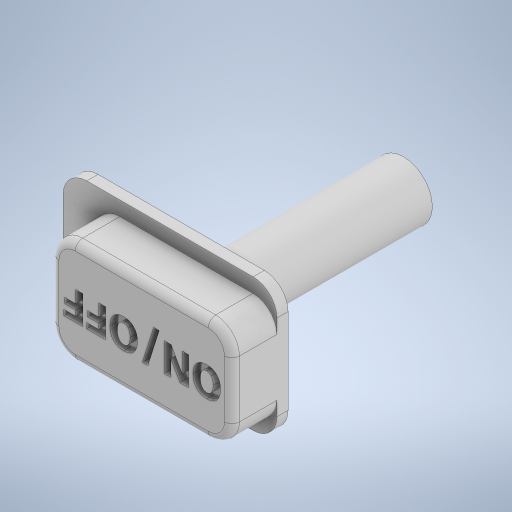
# Autodesk Inventor part: Button Cover
Saved by Autodesk Inventor 2023 (Build 270158000, 158)
## iProperties
Created: 2024-03-21
Part Number: Button Cover
Material: Generic
Document SubType Name: Modeling
Designer: Pobe Tran
Density: 1 g/cm^3
Appearance: Default
Author: Pobe Tran
Autodesk Inventor part; units mm, degrees
ref_plane "YZ Plane" through (0, 0, 0) normal (1, 0, 0) x (0, 1, 0)
ref_plane "XZ Plane" through (0, 0, 0) normal (0, 1, 0) x (-1, 0, 0)
ref_plane "XY Plane" through (0, 0, 0) normal (0, 0, 1) x (1, 0, 0)
sketch "Sketch1" plane through (0, 0, 0) normal (0, 0, 1) x (1, 0, 0)
  circle A0 centre (0, 0) radius 1.75 projected
  circle A1 centre (0, 0) radius 3.85
  point P0 (0, 0)
  constraints: 1 centre point
extrude "Extrusion1" add sketch "Sketch1" against normal blind 5
sketch "Sketch2" plane through (0, 0, 0) normal (0, 0, 1) x (1, 0, 0)
  point P0 (0, 0)
sketch "Sketch3" plane through (0, 0, 0) normal (0, 0, 1) x (1, 0, 0)
  circle A0 centre (0, 0) radius 3.85
  constraints: 1 centre point, 1 coincident
extrude "Extrusion2" add sketch "Sketch3" along normal blind 22.5
sketch "Sketch4" plane through (0, 0, 22.5) normal (0, 0, 1) x (1, 0, 0)
  line L0 (12.065, -6.985) -> (-12.065, -6.985)
  line L1 (-12.065, -6.985) -> (-12.065, 6.985)
  line L2 (-12.065, 6.985) -> (12.065, 6.985)
  line L3 (12.065, 6.985) -> (12.065, -6.985)
  circle A0 centre (0, 0) radius 1.85 projected
  line L4 (12.065, -6.985) -> (-12.065, 6.985) construction
  line L5 (-12.065, -6.985) -> (12.065, 6.985) construction
  line L6 (12.065, 12.065) -> (-12.065, 12.065) construction
  line L7 (-12.065, 12.065) -> (-12.065, 26.035) construction
  line L8 (-12.065, 26.035) -> (12.065, 26.035) construction
  line L9 (12.065, 26.035) -> (12.065, 12.065) construction
  line L10 (12.065, 12.065) -> (-12.065, 26.035) construction
  line L11 (-12.065, 12.065) -> (12.065, 26.035) construction
  line L12 (12.065, -8.89) -> (-16.51, -8.89)
  line L13 (-16.51, -8.89) -> (-16.51, 8.89)
  line L14 (-16.51, 8.89) -> (12.065, 8.89)
  line L15 (16.51, -8.89) -> (-16.51, 8.89) construction
  line L16 (-16.51, -8.89) -> (12.065, 6.4965) construction
  line L17 (12.065, -8.89) -> (12.065, 8.89)
  point P0 (0, 0)
  point P1 (0, 19.05)
  dimension "d6" = 24.13
  dimension "d7" = 13.97
  dimension "d10" = 19.05
  dimension "d16" = 17.78
  constraints: 36 end point, 3 midpoint, 3 parallel, 3 perpendicular, 2 horizontal, 2 point on line, 1 collinear, 1 vertical, 10 other
  measures "d6" distance of L1.end L2.end
  measures "d7" distance of L0.end L1.end
  measures "d10" distance of L0.start L6.start
  measures "d16" distance of L12.end L13.end
extrude "Extrusion3" add sketch "Sketch4" along normal blind 1.5 contours L17 L12 L13 L14 L2 L1 L0 | L0 L1 L2 L3 | A0
extrude "Extrusion4" add sketch "Sketch4" along normal blind 7.5 contours L0 L1 L2 L3 | A0
fillet "Fillet1" radius 3.175 8 edges at (-12.065, 6.985, 27) (12.065, 6.985, 27) (12.065, -6.985, 27) (-12.065, -6.985, 27) (-16.51, -8.89, 23.25) (12.065, 8.89, 23.25) (-16.51, 8.89, 23.25) (12.065, -8.89, 23.25)
sketch "Sketch5" plane through (0, 0, 30) normal (0, 0, 1) x (1, 0, 0)
  line L0 (-12.065, 3.81) -> (-12.065, -3.81) projected
  line L1 (10.7174, -2.4036) -> (-10.7174, -2.4036) construction
  line L2 (-10.7174, -2.4036) -> (-10.7174, 2.4036) construction
  line L3 (-10.7174, 2.4036) -> (10.7174, 2.4036) construction
  line L4 (10.7174, 2.4036) -> (10.7174, -2.4036) construction
  line L5 (-8.89, -6.985) -> (8.89, -6.985) projected
  spline S0 degree 2 poles (6.8549, -0.3288) (6.8549, 0.5974) (7.8429, 1.6565) (8.7013, 1.6565) knots 0 0 0 1 2 2 2
  spline S1 degree 2 poles (8.7013, 1.6565) (9.5627, 1.6565) (10.5445, 0.5851) (10.5445, -0.3288) knots 0 0 0 1 2 2 2
  spline S2 degree 2 poles (10.5445, -0.3288) (10.5445, -1.2458) (9.5627, -2.3141) (8.7013, -2.3141) knots 0 0 0 1 2 2 2
  spline S3 degree 2 poles (8.7013, -2.3141) (7.8429, -2.3141) (6.8549, -1.252) (6.8549, -0.3288) knots 0 0 0 1 2 2 2
  spline S4 degree 2 poles (7.8429, -0.3288) (7.8429, -0.6715) (7.9819, -1.1501) (8.1023, -1.3014) knots 0 0 0 1 2 2 2
  spline S5 degree 2 poles (8.1023, -1.3014) (8.2227, -1.4589) (8.5315, -1.5947) (8.6982, -1.5947) knots 0 0 0 1 2 2 2
  spline S6 degree 2 poles (8.6982, -1.5947) (8.8742, -1.5947) (9.1613, -1.4681) (9.2941, -1.3076) knots 0 0 0 1 2 2 2
  spline S7 degree 2 poles (9.2941, -1.3076) (9.4114, -1.1594) (9.5565, -0.6684) (9.5565, -0.3288) knots 0 0 0 1 2 2 2
  spline S8 degree 2 poles (9.5565, -0.3288) (9.5565, 0.0232) (9.4176, 0.4863) (9.2972, 0.6437) knots 0 0 0 1 2 2 2
  spline S9 degree 2 poles (9.2972, 0.6437) (9.1768, 0.8012) (8.8649, 0.9371) (8.6982, 0.9371) knots 0 0 0 1 2 2 2
  spline S10 degree 2 poles (8.6982, 0.9371) (8.5284, 0.9371) (8.2134, 0.7919) (8.0992, 0.6376) knots 0 0 0 1 2 2 2
  spline S11 degree 2 poles (8.0992, 0.6376) (7.9757, 0.4708) (7.8429, 0.0293) (7.8429, -0.3288) knots 0 0 0 1 2 2 2
  line L6 (3.0233, 1.5762) -> (3.9434, 1.5762)
  line L7 (3.9434, 1.5762) -> (5.4131, -1.0791)
  line L8 (5.4131, -1.0791) -> (5.4131, 1.5762)
  line L9 (5.4131, 1.5762) -> (6.2868, 1.5762)
  line L10 (6.2868, 1.5762) -> (6.2868, -2.2338)
  line L11 (6.2868, -2.2338) -> (5.1136, -2.2338)
  line L12 (5.1136, -2.2338) -> (3.8971, -0.0509)
  line L13 (3.8971, -0.0509) -> (3.8971, -2.2338)
  line L14 (3.8971, -2.2338) -> (3.0233, -2.2338)
  line L15 (3.0233, -2.2338) -> (3.0233, 1.5762)
  line L16 (0.0902, -2.4036) -> (1.6062, 2.4036)
  line L17 (1.6062, 2.4036) -> (2.341, 2.4036)
  line L18 (2.341, 2.4036) -> (0.8281, -2.4036)
  line L19 (0.8281, -2.4036) -> (0.0902, -2.4036)
  spline S12 degree 2 poles (-4.2416, -0.3288) (-4.2416, 0.5974) (-3.2536, 1.6565) (-2.3953, 1.6565) knots 0 0 0 1 2 2 2
  spline S13 degree 2 poles (-2.3953, 1.6565) (-1.5339, 1.6565) (-0.552, 0.5851) (-0.552, -0.3288) knots 0 0 0 1 2 2 2
  spline S14 degree 2 poles (-0.552, -0.3288) (-0.552, -1.2458) (-1.5339, -2.3141) (-2.3953, -2.3141) knots 0 0 0 1 2 2 2
  spline S15 degree 2 poles (-2.3953, -2.3141) (-3.2536, -2.3141) (-4.2416, -1.252) (-4.2416, -0.3288) knots 0 0 0 1 2 2 2
  spline S16 degree 2 poles (-3.2536, -0.3288) (-3.2536, -0.6715) (-3.1147, -1.1501) (-2.9943, -1.3014) knots 0 0 0 1 2 2 2
  spline S17 degree 2 poles (-2.9943, -1.3014) (-2.8738, -1.4589) (-2.5651, -1.5947) (-2.3984, -1.5947) knots 0 0 0 1 2 2 2
  spline S18 degree 2 poles (-2.3984, -1.5947) (-2.2224, -1.5947) (-1.9352, -1.4681) (-1.8025, -1.3076) knots 0 0 0 1 2 2 2
  spline S19 degree 2 poles (-1.8025, -1.3076) (-1.6851, -1.1594) (-1.54, -0.6684) (-1.54, -0.3288) knots 0 0 0 1 2 2 2
  spline S20 degree 2 poles (-1.54, -0.3288) (-1.54, 0.0232) (-1.679, 0.4863) (-1.7994, 0.6437) knots 0 0 0 1 2 2 2
  spline S21 degree 2 poles (-1.7994, 0.6437) (-1.9198, 0.8012) (-2.2316, 0.9371) (-2.3984, 0.9371) knots 0 0 0 1 2 2 2
  spline S22 degree 2 poles (-2.3984, 0.9371) (-2.5682, 0.9371) (-2.8831, 0.7919) (-2.9973, 0.6376) knots 0 0 0 1 2 2 2
  spline S23 degree 2 poles (-2.9973, 0.6376) (-3.1208, 0.4708) (-3.2536, 0.0293) (-3.2536, -0.3288) knots 0 0 0 1 2 2 2
  line L20 (-7.36, -1.5083) -> (-5.7607, -1.5083)
  line L21 (-5.7607, -1.5083) -> (-5.7607, -0.7889)
  line L22 (-5.7607, -0.7889) -> (-7.2334, -0.7889)
  line L23 (-7.2334, -0.7889) -> (-7.2334, -0.0633)
  line L24 (-7.2334, -0.0633) -> (-5.7607, -0.0633)
  line L25 (-5.7607, -0.0633) -> (-5.7607, 1.5762)
  line L26 (-5.7607, 1.5762) -> (-4.8097, 1.5762)
  line L27 (-4.8097, 1.5762) -> (-4.8097, -2.2338)
  line L28 (-4.8097, -2.2338) -> (-7.36, -2.2338)
  line L29 (-7.36, -2.2338) -> (-7.36, -1.5083)
  line L30 (-10.4043, -1.5083) -> (-8.805, -1.5083)
  line L31 (-8.805, -1.5083) -> (-8.805, -0.7889)
  line L32 (-8.805, -0.7889) -> (-10.2777, -0.7889)
  line L33 (-10.2777, -0.7889) -> (-10.2777, -0.0633)
  line L34 (-10.2777, -0.0633) -> (-8.805, -0.0633)
  line L35 (-8.805, -0.0633) -> (-8.805, 1.5762)
  line L36 (-8.805, 1.5762) -> (-7.854, 1.5762)
  line L37 (-7.854, 1.5762) -> (-7.854, -2.2338)
  line L38 (-7.854, -2.2338) -> (-10.4043, -2.2338)
  line L39 (-10.4043, -2.2338) -> (-10.4043, -1.5083)
  point P0 (0, 0)
  point P1 (-9.9875, 0)
  point P2 (-12.065, 0)
  point P3 (-0.3598, 2.5871)
  point P4 (-10.7174, 0)
  point P5 (-12.065, 0)
  point P6 (0, -2.4036)
  point P7 (0, -6.985)
  constraints: 5 midpoint, 2 horizontal alignment, 1 vertical alignment, 2 other
emboss "Emboss1" sketch "Sketch5" operation cut depth 1 direction (0, 0, -1)
fillet "Fillet2" radius 1 8 edges at (-11.1351, 6.0551, 30) (-12.065, 0, 30) (-11.1351, -6.0551, 30) (0, -6.985, 30) (11.1351, -6.0551, 30) (12.065, 0, 30) (11.1351, 6.0551, 30) (0, 6.985, 30)
body "Solid1"
